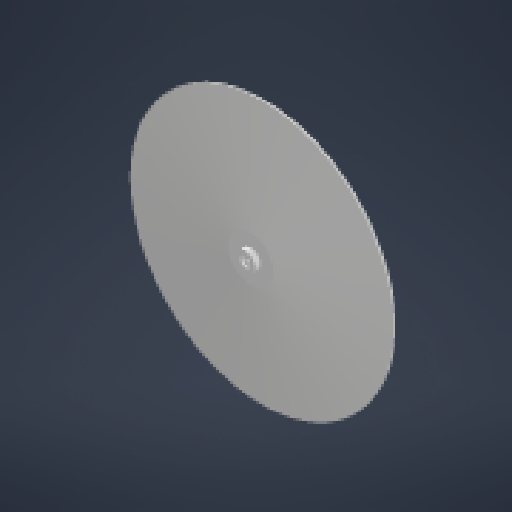
# Autodesk Inventor part: center_disk
Saved by Autodesk Inventor 2026 (Build 300175050, 175E)
## iProperties
Created: 2026-05-09
Part Number: center_disk
Material: Generic
Document SubType Name: Modeling
Designer: sniel
Density: 1 g/cm^3
Appearance: Default
Author: sniel
Autodesk Inventor part; units mm, degrees
ref_plane "YZ Plane" through (0, 0, 0) normal (1, 0, 0) x (0, 1, 0)
ref_plane "XZ Plane" through (0, 0, 0) normal (0, 1, 0) x (-1, 0, 0)
ref_plane "XY Plane" through (0, 0, 0) normal (0, 0, 1) x (1, 0, 0)
sketch "Sketch1" plane through (0, 0, 0) normal (0, 0, 1) x (1, 0, 0)
  arc A0 (-1.9795, 6.7143) -> (1.9795, 6.7143) centre (0, 7) ccw
  arc A1 (-1.9795, 6.7143) -> (-1.9795, -6.7143) centre (0, 0) ccw
  arc A2 (1.9795, -6.7143) -> (-1.9795, -6.7143) centre (0, -7) ccw
  arc A3 (1.9795, -6.7143) -> (1.9795, 6.7143) centre (0, 0) ccw
  line L0 (3.6, 1.9621) -> (3.6, -1.9621)
  arc A4 (3.6, 1.9621) -> (3.6, -1.9621) centre (0, 0) ccw
  circle A5 centre (0, -7) radius 1.75
  circle A6 centre (0, 7) radius 1.75
  circle A7 centre (0, 0) radius 7.5
  circle A8 centre (0, 0) radius 102.5
  point P0 (0, 0)
  point P1 (-1.7242, 7.2991)
  point P2 (1.7242, 7.2991)
  point P3 (1.7242, -7.2991)
  point P4 (-1.7242, -7.2991)
  dimension "d0" = 3.5
  dimension "d1" = 3.5
  dimension "d2" = 15
  dimension "d3" = 205
  constraints: 10 point on circle, 9 centre point, 4 coincident, 2 end point
  measures "d0" diameter of A5
  measures "d1" diameter of A6
  measures "d2" diameter of A7
  measures "d3" diameter of A8
extrude "Extrusion1" add sketch "Sketch1" against normal blind 8.25 contours A5 A7 | A7 A5 | A7 A6 | A6 A7 | A8
fillet "Fillet1" radius 3.5 1 edges at (-102.5, 0, -8.25)
sketch "Sketch2" plane through (0, 0, 0) normal (0, 0, 1) x (1, 0, 0)
  circle A0 centre (0, 0) radius 5.25
  arc A1 (1.7242, -7.2991) -> (-1.7242, -7.2991) centre (0, -7) ccw
  circle A2 centre (0, 0) radius 10
  circle A3 centre (0, 0) radius 102.5
  dimension "d7" = 20
  constraints: 4 centre point, 2 coincident, 2 point on circle
  measures "d7" diameter of A2
extrude "Extrusion2" add sketch "Sketch2" along normal blind 4 contours A2 | A3
sketch "Sketch3" plane through (0, 0, 4) normal (0, 0, 1) x (1, 0, 0)
  circle A0 centre (0, 0) radius 5.25
  arc A1 (1.7242, -7.2991) -> (1.7242, 7.2991) centre (0, 0) ccw
  circle A2 centre (0, 0) radius 1.4142
  circle A3 centre (0, 0) radius 3.6056
  arc A4 (0, -5.25) -> (0, 5.25) centre (0, 0) ccw
  arc A5 (1.7242, -7.2991) -> (1.7242, 7.2991) centre (0, 0) ccw
  circle A6 centre (0, 0) radius 7.5
  point P0 (1.7242, 7.2991)
  constraints: 6 centre point, 6 point on circle, 4 coincident, 3 other
extrude "Extrusion3" add sketch "Sketch3" along normal blind 4 contours A0 | A6 A1 | A3
sketch "Sketch4" plane through (0, 0, 8) normal (0, 0, 1) x (1, 0, 0)
  circle A0 centre (0, 0) radius 4
  constraints: 1 centre point, 1 coincident
extrude "Extrusion4" cut sketch "Sketch4" against normal blind 2
sketch "Sketch5" plane through (0, 0, 0) normal (1, 0, 0) x (0, 1, 0)
  line L0 (102.5, 4) -> (-102.5, 4)
  line L1 (-102.5, -4.75) -> (102.5, -4.75)
  line L2 (7.5, 8) -> (-7.5, 8)
  line L3 (-7.5, 4) -> (7.5, 4)
  line L4 (7.5, 4) -> (17.5, 4)
  line L5 (17.5, 4) -> (102.5, -4.75)
  line L6 (102.5, -4.75) -> (102.5, 16)
  line L7 (102.5, 16) -> (7.5, 16)
  line L8 (7.5, 16) -> (7.5, 4)
  line L9 (0, -13.1) -> (0, 20.85) projected
  point P0 (0, 0)
  dimension "d14" = 10
  constraints: 18 end point, 2 perpendicular, 1 point on line, 1 vertical
  measures "d14" distance of L3.end L4.end
revolve "Revolution1" cut sketch "Sketch5" angle 360 about axis through (0, 0, -10) along (0, 0, 1) contours L6 L5 L0 | L0 L8 L7 L6
body "Solid1"
